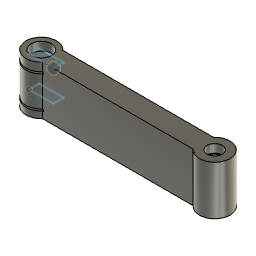
ペン側腕(高) v1 (Autodesk Fusion 360 design; units mm, degrees)
Autodesk Fusion 360 part; units mm, degrees
note: some values were not read from the file. Set by a fixed rule: which sketch regions a step uses.
sketch "スケッチ1" plane through (0, 0, 0) normal (0, 0, 1) x (1, 0, 0)
  line L0 (0, 0) -> (85, 0)
  line L1 (85, 0) -> (85, 10)
  line L2 (85, 10) -> (0, 10)
  line L3 (0, 10) -> (0, 0)
  circle A0 centre (85, 5) radius 7.5
  circle A1 centre (0, 5) radius 7.5
  dimension "d1" = 10
  dimension "d2" = 15
  dimension "d3" = 15
  constraint horizontal L0
  constraint vertical L1
  constraint horizontal L2
  constraint vertical L3
  constraint coincident L0.start L3.end
  constraint midpoint L1 A0.centre
  constraint midpoint L3 A1.centre
  measures "d1" distance of L0.start L2.end
  measures "d2" diameter of A0
  measures "d3" diameter of A1
extrude "押し出し1" add sketch "スケッチ1" along normal blind 24
sketch "スケッチ2" plane through (0, 0, 24) normal (0, 0, 1) x (-1, 0, 0)
  line L0 (-79.4098, -10) -> (-5.5902, -10)
  arc A0 (-5.5902, -10) -> (-5.5902, 0) centre (0, -5) ccw
  line L1 (-5.5902, 0) -> (-79.4098, 0)
  arc A1 (-79.4098, 0) -> (-79.4098, -10) centre (-85, -5) ccw
  circle A2 centre (-85, -5) radius 3.75
  dimension "d6" = 7.5
  constraint concentric A1 A2
  measures "d6" diameter of A2
extrude "押し出し2" cut sketch "スケッチ2" against normal blind 4.1 contours A2
sketch "スケッチ3" plane through (0, 0, 19.9) normal (0, 0, 1) x (-1, 0, 0)
  circle A0 centre (-85, -5) radius 3.75
  circle A1 centre (-85, -5) radius 3.3
  dimension "d9" = 6.6
  constraint concentric A0 A1
  measures "d9" diameter of A1
extrude "押し出し3" cut sketch "スケッチ3" against normal blind 1.9 contours A1
sketch "スケッチ4" plane through (0, 0, 0) normal (0, 0, -1) x (1, 0, 0)
  line L0 (5.5902, -10) -> (79.4098, -10)
  arc A0 (79.4098, -10) -> (79.4098, 0) centre (85, -5) ccw
  line L1 (79.4098, 0) -> (5.5902, 0)
  arc A1 (5.5902, 0) -> (5.5902, -10) centre (0, -5) ccw
  circle A2 centre (85, -5) radius 2.25
  dimension "d12" = 4.5
  constraint concentric A0 A2
  measures "d12" diameter of A2
extrude "押し出し4" cut sketch "スケッチ4" against normal blind 5.8 contours A2
sketch "スケッチ5" plane through (0, 0, 5.8) normal (0, 0, -1) x (1, 0, 0)
  circle A0 centre (85, -5) radius 2.25
  circle A1 centre (85, -5) radius 1.7
  dimension "d15" = 3.4
  constraint concentric A0 A1
  measures "d15" diameter of A1
extrude "押し出し5" cut sketch "スケッチ5" against normal blind 13 contours A1
sketch "スケッチ6" plane through (0, 0, 0) normal (0, 0, 1) x (1, 0, 0)
  circle A0 centre (0, 5) radius 5
  dimension "d18" = 10
  measures "d18" diameter of A0
extrude "押し出し6" cut sketch "スケッチ6" along normal blind 4.1
sketch "スケッチ7" plane through (0, 0, 4.1) normal (0, 0, -1) x (1, 0, 0)
  circle A0 centre (0, -5) radius 5
  circle A1 centre (0, -5) radius 6
  dimension "d21" = 12
  constraint concentric A0 A1
  measures "d21" diameter of A1
extrude "押し出し7" cut sketch "スケッチ7" along normal blind 0.85 contours A0 | A1
sketch "スケッチ8" plane through (0, 0, 24) normal (0, 0, 1) x (-1, 0, 0)
  circle A0 centre (-85, -5) radius 3.75
  line L0 (-79.4098, -10) -> (-5.5902, -10)
  arc A1 (-5.5902, -10) -> (-5.5902, 0) centre (0, -5) ccw
  line L1 (-5.5902, 0) -> (-79.4098, 0)
  arc A2 (-79.4098, 0) -> (-79.4098, -10) centre (-85, -5) ccw
  circle A3 centre (0, -5) radius 5
  dimension "d24" = 10
  constraint concentric A1 A3
  measures "d24" diameter of A3
extrude "押し出し8" cut sketch "スケッチ8" against normal blind 4.1 contours A3
sketch "スケッチ9" plane through (0, 0, 19.9) normal (0, 0, 1) x (-1, 0, 0)
  circle A0 centre (0, -5) radius 5
  circle A1 centre (0, -5) radius 6
  dimension "d27" = 12
  constraint concentric A0 A1
  measures "d27" diameter of A1
extrude "押し出し9" cut sketch "スケッチ9" against normal blind 0.85 contours A0 | A1
sketch "スケッチ10" plane through (0, 0, 19.05) normal (0, 0, 1) x (-1, 0, 0)
  circle A0 centre (0, -5) radius 6
  line L0 (-6, -5) -> (6, -5)
  line L1 (6, -5) -> (6, -10)
  line L2 (6, -10) -> (-6, -10)
  line L3 (-6, -10) -> (-6, -5)
  constraint horizontal L0
  constraint vertical L1
  constraint horizontal L2
  constraint vertical L3
  constraint coincident A0 L0.start
sketch "スケッチ11" plane through (0, 0, 0) normal (0, 1, 0) x (1, 0, 0)
  line L0 (6, -19.05) -> (-6.0119, -19.05)
  line L1 (-6.0119, -19.05) -> (-6.0119, -19.9)
  line L2 (-6.0119, -19.9) -> (6, -19.9)
  line L3 (6, -19.9) -> (6, -19.05)
  dimension "d30" = 0.85
  constraint horizontal L0
  constraint vertical L1
  constraint horizontal L2
  constraint vertical L3
  measures "d30" distance of L0.start L2.end
extrude "押し出し10" cut sketch "スケッチ11" against normal blind 2.5
sketch "スケッチ12" plane through (0, 0, 0) normal (0, -1, 0) x (1, 0, 0)
  line L0 (-3.3166, 19.05) -> (-3.3166, 19.9)
  line L1 (-3.3166, 19.9) -> (-5.5902, 19.9)
  line L2 (-5.5902, 19.9) -> (-5.5902, 19.05)
  line L3 (-5.5902, 19.05) -> (-3.3166, 19.05)
sketch "スケッチ13" plane through (0, 0, 0) normal (0, -1, 0) x (1, 0, 0)
  line L0 (5.5902, 19.05) -> (5.5902, 0)
  line L1 (5.5902, 0) -> (79.4098, 0)
  line L2 (79.4098, 0) -> (79.4098, 24)
  line L3 (79.4098, 24) -> (5.5902, 24)
  line L4 (5.5902, 24) -> (5.5902, 19.9)
  line L5 (5.5902, 19.9) -> (3.3166, 19.9)
  line L6 (3.3166, 19.9) -> (3.3166, 19.05)
  line L7 (3.3166, 19.05) -> (5.5902, 19.05)
  line L8 (6, 19.05) -> (3.3166, 19.05)
  line L9 (3.3166, 19.05) -> (3.3166, 19.9)
  line L10 (3.3166, 19.9) -> (6, 19.9)
  line L11 (6, 19.9) -> (6, 19.05)
  constraint horizontal L8
  constraint vertical L9
  constraint horizontal L10
  constraint vertical L11
  constraint coincident L5.end L6.start
sketch "スケッチ14" plane through (0, 0, 0) normal (0, -1, 0) x (1, 0, 0)
  line L0 (-6, 19.05) -> (-3.3174, 19.05)
  line L1 (-3.3174, 19.05) -> (-3.3174, 19.8997)
  line L2 (-3.3174, 19.8997) -> (-6, 19.8997)
  line L3 (-6, 19.8997) -> (-6, 19.05)
  constraint horizontal L0
  constraint vertical L1
  constraint horizontal L2
  constraint vertical L3
extrude "押し出し11" cut sketch "スケッチ13" sketch "スケッチ14" against normal blind 5 contours L5 L6 L7 L8 L9 L10 L11 of sketch 2
sketch "スケッチ15" plane through (0, 0, 4.1) normal (0, 0, -1) x (1, 0, 0)
  circle A0 centre (0, -5) radius 6
  line L0 (-6, -5) -> (6, -5)
  line L1 (6, -5) -> (6, -10)
  line L2 (6, -10) -> (-6, -10)
  line L3 (-6, -10) -> (-6, -5)
  constraint horizontal L0
  constraint vertical L1
  constraint horizontal L2
  constraint vertical L3
  constraint coincident A0 L0.start
sketch "スケッチ16" plane through (0, 0, 0) normal (0, 1, 0) x (1, 0, 0)
  line L0 (-6, -4.1) -> (6.0025, -4.1)
  line L1 (6.0025, -4.1) -> (6.0025, -3.25)
  line L2 (6.0025, -3.25) -> (-6, -3.25)
  line L3 (-6, -3.25) -> (-6, -4.1)
  dimension "d35" = 0.85
  constraint horizontal L0
  constraint vertical L1
  constraint horizontal L2
  constraint vertical L3
  measures "d35" distance of L0.start L2.end
extrude "押し出し12" cut sketch "スケッチ16" against normal blind 2.5
sketch "スケッチ17" plane through (0, 0, 0) normal (0, -1, 0) x (1, 0, 0)
  line L0 (5.5902, 3.25) -> (5.5902, 0)
  line L1 (5.5902, 0) -> (79.4098, 0)
  line L2 (79.4098, 0) -> (79.4098, 24)
  line L3 (79.4098, 24) -> (5.5902, 24)
  line L4 (5.5902, 24) -> (5.5902, 19.9)
  line L5 (5.5902, 19.9) -> (6, 19.9)
  line L6 (6, 19.9) -> (6, 19.05)
  line L7 (6, 19.05) -> (5.5902, 19.05)
  line L8 (5.5902, 19.05) -> (5.5902, 4.1)
  line L9 (5.5902, 4.1) -> (3.3166, 4.1)
  line L10 (3.3166, 4.1) -> (3.3166, 3.25)
  line L11 (3.3166, 3.25) -> (5.5902, 3.25)
  line L12 (6, 4.1) -> (3.3166, 4.1)
  line L13 (3.3166, 4.1) -> (3.3166, 3.25)
  line L14 (3.3166, 3.25) -> (6, 3.25)
  line L15 (6, 3.25) -> (6, 4.1)
  line L16 (-6, 4.1) -> (-3.3175, 4.1)
  line L17 (-3.3175, 4.1) -> (-3.3175, 3.25)
  line L18 (-3.3175, 3.25) -> (-6, 3.25)
  line L19 (-6, 3.25) -> (-6, 4.1)
  constraint horizontal L12
  constraint vertical L13
  constraint horizontal L14
  constraint vertical L15
  constraint coincident L10.end L11.start
  constraint horizontal L16
  constraint vertical L17
  constraint horizontal L18
  constraint vertical L19
extrude "押し出し13" cut sketch "スケッチ17" against normal blind 5 contours L9 L10 L11 L12 L13 L14 L15 | L16 L17 L18 L19
sketch "スケッチ18" plane through (0, 0, 4.1) normal (0, 0, -1) x (1, 0, 0)
  circle A0 centre (0, -5) radius 1.7
  dimension "d40" = 3.4
  measures "d40" diameter of A0
extrude "押し出し14" cut sketch "スケッチ18" against normal blind 15
